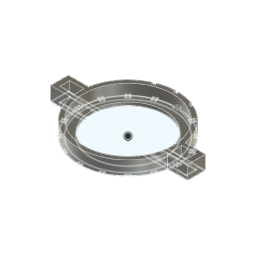
filter holder v6 (Autodesk Fusion 360 design; units mm, degrees)
Autodesk Fusion 360 part; units mm, degrees
sketch "Sketch1" plane through (0, 0, 0) normal (0, 0, 1) x (1, 0, 0)
  circle A0 centre (0, 0) radius 12.775
  circle A1 centre (0, 0) radius 14
  circle A2 centre (0, 0) radius 10.5
  line L0 (19.5, 2.5) -> (-19.5, 2.5)
  line L1 (-19.5, 2.5) -> (-19.5, -2.5)
  line L2 (-19.5, -2.5) -> (19.5, -2.5)
  line L3 (19.5, -2.5) -> (19.5, 2.5)
  line L4 (19.5, 2.5) -> (-19.5, -2.5) construction
  line L5 (-19.5, 2.5) -> (19.5, -2.5) construction
  line L6 (18, -1.4) -> (-18, -1.4)
  line L7 (-18, -1.4) -> (-18, 1.4)
  line L8 (-18, 1.4) -> (18, 1.4)
  line L9 (18, 1.4) -> (18, -1.4)
  line L10 (18, -1.4) -> (-18, 1.4) construction
  line L11 (-18, -1.4) -> (18, 1.4) construction
  line L12 (0.5, 13.5) -> (-0.5, 13.5)
  line L13 (-0.5, 13.5) -> (-0.5, 14.5)
  line L14 (-0.5, 14.5) -> (0.5, 14.5)
  line L15 (0.5, 14.5) -> (0.5, 13.5)
  line L16 (0.5, 13.5) -> (-0.5, 14.5) construction
  line L17 (-0.5, 13.5) -> (0.5, 14.5) construction
  line L18 (-4.7043, 12.6637) -> (-5.6282, 12.281)
  line L19 (-5.6282, 12.281) -> (-6.0108, 13.2049)
  line L20 (-6.0108, 13.2049) -> (-5.087, 13.5876)
  line L21 (-5.087, 13.5876) -> (-4.7043, 12.6637)
  line L22 (-9.1924, 9.8995) -> (-9.8995, 9.1924)
  line L23 (-9.8995, 9.1924) -> (-10.6066, 9.8995)
  line L24 (-10.6066, 9.8995) -> (-9.8995, 10.6066)
  line L25 (-9.8995, 10.6066) -> (-9.1924, 9.8995)
  line L26 (-12.281, 5.6282) -> (-12.6637, 4.7043)
  line L27 (-12.6637, 4.7043) -> (-13.5876, 5.087)
  line L28 (-13.5876, 5.087) -> (-13.2049, 6.0108)
  line L29 (-13.2049, 6.0108) -> (-12.281, 5.6282)
  line L30 (-13.5, 0.5) -> (-13.5, -0.5)
  line L31 (-13.5, -0.5) -> (-14.5, -0.5)
  line L32 (-14.5, -0.5) -> (-14.5, 0.5)
  line L33 (-14.5, 0.5) -> (-13.5, 0.5)
  line L34 (-12.6637, -4.7043) -> (-12.281, -5.6282)
  line L35 (-12.281, -5.6282) -> (-13.2049, -6.0108)
  line L36 (-13.2049, -6.0108) -> (-13.5876, -5.087)
  line L37 (-13.5876, -5.087) -> (-12.6637, -4.7043)
  line L38 (-9.8995, -9.1924) -> (-9.1924, -9.8995)
  line L39 (-9.1924, -9.8995) -> (-9.8995, -10.6066)
  line L40 (-9.8995, -10.6066) -> (-10.6066, -9.8995)
  line L41 (-10.6066, -9.8995) -> (-9.8995, -9.1924)
  line L42 (-5.6282, -12.281) -> (-4.7043, -12.6637)
  line L43 (-4.7043, -12.6637) -> (-5.087, -13.5876)
  line L44 (-5.087, -13.5876) -> (-6.0108, -13.2049)
  line L45 (-6.0108, -13.2049) -> (-5.6282, -12.281)
  line L46 (-0.5, -13.5) -> (0.5, -13.5)
  line L47 (0.5, -13.5) -> (0.5, -14.5)
  line L48 (0.5, -14.5) -> (-0.5, -14.5)
  line L49 (-0.5, -14.5) -> (-0.5, -13.5)
  line L50 (4.7043, -12.6637) -> (5.6282, -12.281)
  line L51 (5.6282, -12.281) -> (6.0108, -13.2049)
  line L52 (6.0108, -13.2049) -> (5.087, -13.5876)
  line L53 (5.087, -13.5876) -> (4.7043, -12.6637)
  line L54 (9.1924, -9.8995) -> (9.8995, -9.1924)
  line L55 (9.8995, -9.1924) -> (10.6066, -9.8995)
  line L56 (10.6066, -9.8995) -> (9.8995, -10.6066)
  line L57 (9.8995, -10.6066) -> (9.1924, -9.8995)
  line L58 (12.281, -5.6282) -> (12.6637, -4.7043)
  line L59 (12.6637, -4.7043) -> (13.5876, -5.087)
  line L60 (13.5876, -5.087) -> (13.2049, -6.0108)
  line L61 (13.2049, -6.0108) -> (12.281, -5.6282)
  line L62 (13.5, -0.5) -> (13.5, 0.5)
  line L63 (13.5, 0.5) -> (14.5, 0.5)
  line L64 (14.5, 0.5) -> (14.5, -0.5)
  line L65 (14.5, -0.5) -> (13.5, -0.5)
  line L66 (12.6637, 4.7043) -> (12.281, 5.6282)
  line L67 (12.281, 5.6282) -> (13.2049, 6.0108)
  line L68 (13.2049, 6.0108) -> (13.5876, 5.087)
  line L69 (13.5876, 5.087) -> (12.6637, 4.7043)
  line L70 (9.8995, 9.1924) -> (9.1924, 9.8995)
  line L71 (9.1924, 9.8995) -> (9.8995, 10.6066)
  line L72 (9.8995, 10.6066) -> (10.6066, 9.8995)
  line L73 (10.6066, 9.8995) -> (9.8995, 9.1924)
  line L74 (5.6282, 12.281) -> (4.7043, 12.6637)
  line L75 (4.7043, 12.6637) -> (5.087, 13.5876)
  line L76 (5.087, 13.5876) -> (6.0108, 13.2049)
  line L77 (6.0108, 13.2049) -> (5.6282, 12.281)
  point P0 (0, 14)
  dimension "d3" = 25.55
  dimension "d4" = 28
  dimension "d5" = 21
  dimension "d10" = 39
  dimension "d11" = 5
  dimension "d12" = 36
  dimension "d13" = 2.8
  dimension "d16" = 1
  dimension "d17" = 1
  dimension "d21" = 360
  constraint coincident A0.centre A1.centre
  constraint horizontal L0
  constraint perpendicular L0 L1
  constraint parallel L0 L2
  constraint parallel L1 L3
  constraint coincident L4 A0.centre
  constraint coincident L5 A0.centre
  constraint horizontal L6
  constraint perpendicular L6 L7
  constraint parallel L6 L8
  constraint parallel L7 L9
  constraint coincident L10 A0.centre
  constraint coincident L11 A0.centre
  constraint horizontal L12
  constraint perpendicular L12 L13
  constraint parallel L12 L14
  constraint parallel L13 L15
  constraint coincident L16 P0
  constraint coincident L17 P0
  constraint coincident A1 P0
  measures "d3" diameter of A0
  measures "d4" diameter of A1
  measures "d5" diameter of A2
  measures "d10" distance of L1.end L2.end
  measures "d11" distance of L0.end L1.end
  measures "d12" distance of L7.end L8.end
  measures "d13" distance of L6.end L7.end
  measures "d16" distance of L13.end L14.end
  measures "d17" distance of L12.end L13.end
extrude "Extrude2" add sketch "Sketch1" along normal blind 2 contours A0 A1 L6 L8 L62 L63 L65 | A0 A1 L0 L8 | A0 A1 L2 L6 | A0 A1 L0 L12 L13 L15 L18 L19 L21 L22 L23 L25 L26 L27 L29 L66 L67 L69 L70 L71 L73 L74 L75 L77 | A0 A1 L2 L34 L35 L37 L38 L39 L41 L42 L43 L45 L46 L47 L49 L50 L51 L53 L54 L55 L57 L58 L59 L61 | A0 A1 L0 L8 | A1 L62 L63 L65 | A0 A1 L2 L6 | A0 A1 L6 L8 L30 L31 L33 | A1 L66 L67 L69 | A1 L58 L59 L61 | A1 L26 L27 L29 | A1 L34 L35 L37 | A1 L30 L31 L33 | A1 L70 L71 L73 | A1 L54 L55 L57 | A1 L22 L23 L25 | A1 L38 L39 L41 | A1 L74 L75 L77 | A1 L50 L51 L53 | A1 L18 L19 L21 | A1 L42 L43 L45 | A1 L12 L13 L15 | A1 L46 L47 L49 makes body 1
extrude "Extrude1" add sketch "Sketch1" along normal blind 1 separate body contours A0 A2 L6 L8 | A0 A2 L0 L8 | A0 A2 L2 L6 | A0 A2 L0 | A0 A2 L2 | A0 A2 L0 L8 | A0 A2 L6 L8 | A0 A2 L2 L6 makes body 2
extrude "Extrude3" add sketch "Sketch1" along normal blind 4 contours A1 L0 L2 L3 L6 L8 L9 | A1 L0 L1 L2 L6 L7 L8 bodies 1
extrude "Extrude4" cut sketch "Sketch1" along normal blind 4.762 contours A1 L12 L13 L15 bodies 1
extrude "Extrude5" cut sketch "Sketch1" along normal blind 6.934 contours A1 L70 L71 L73 | A1 L74 L75 L77 | A1 L18 L19 L21 bodies 1
extrude "Extrude6" add 1 faces at (-1.93, 13.0172, 2) along direction (0, 0, 1) blind 2 on bodies 1 bodies 1
